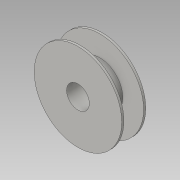
# Autodesk Inventor part: Spool Colorfabb
Saved by Autodesk Inventor 2016 (Build 200138000, 138)
## iProperties
Created: 2017-05-19
Part Number: Spool Colorfabb
Material: Generic
Document SubType Name: Modeling
Designer: 31745
Density: 1 g/cm^3
Appearance: Default
Author: 31745
Autodesk Inventor part; units mm, degrees
ref_plane "YZ Plane" through (0, 0, 0) normal (1, 0, 0) x (0, 1, 0)
ref_plane "XZ Plane" through (0, 0, 0) normal (0, 1, 0) x (-1, 0, 0)
ref_plane "XY Plane" through (0, 0, 0) normal (0, 0, 1) x (1, 0, 0)
sketch "Sketch1" plane through (0, 0, 0) normal (0, 0, 1) x (1, 0, 0)
  line L0 (0, 0) -> (100, 0)
  line L1 (100, 0) -> (100, 5)
  line L2 (100, 5) -> (52.5, 5)
  line L3 (0, 19.2579) -> (0, 78.5591)
  line L4 (52.5, 50) -> (100, 50)
  line L5 (100, 50) -> (100, 55)
  line L6 (100, 55) -> (26, 55)
  line L7 (0, 102.6022) -> (0, 0)
  line L8 (52.5, 50) -> (52.5, 5)
  line L9 (26, 55) -> (26, 0)
  dimension "d0" = 26
  dimension "d1" = 52.5
  dimension "d2" = 100
  dimension "d3" = 45
  dimension "d4" = 55
  dimension "d5" = 5
  constraints: 20 end point, 5 perpendicular, 2 parallel, 2 point on line, 2 vertical, 1 horizontal, 1 vertical alignment
  measures "d0" distance between parallel lines of L3 L9
  measures "d1" distance between parallel lines of L3 L8
  measures "d2" distance between parallel lines of L3 L5
  measures "d3" distance of L4.start L2.end
  measures "d4" distance between parallel lines of L0 L6
  measures "d5" distance between parallel lines of L0 L2
revolve "Revolution1" add sketch "Sketch1" angle 360 about axis through (0, 19.2579, 0) along (0, 1, 0)
body "Solid1"
